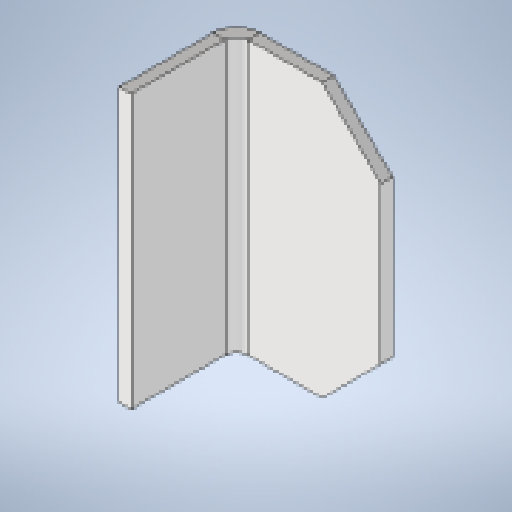
# Autodesk Inventor part: PNS-0812 floor ring  strengthen
Saved by Autodesk Inventor 2025.1 (Build 291241020, 241B)
## iProperties
Created: 2024-05-23
Part Number: PNS-0812 floor ring  strengthen
Material: Generic
Document SubType Name: Sheet Metal
Designer: user
Mass: 0.559799 g
Surface Area: 23.3947 cm^2
Volume: 0.559799 cm^3
Density: 1 g/cm^3
Flat Pattern Width: 12.9572 cm
Flat Pattern Length: 14 cm
Flat Pattern Area: 181.4 cm^2
Sheet Metal Rule: Default_mm
Sheet Metal Width: 129.572 mm
Sheet Metal Length: 140.000 mm
Sheet Metal Area: 18140.035 mm^2
Appearance: Default
Author: admin
Autodesk Inventor part; units mm, degrees
ref_plane "YZ Plane" through (0, 0, 0) normal (1, 0, 0) x (0, 1, 0)
ref_plane "XZ Plane" through (0, 0, 0) normal (0, 1, 0) x (-1, 0, 0)
ref_plane "XY Plane" through (0, 0, 0) normal (0, 0, 1) x (1, 0, 0)
sketch "Sketch1" plane through (0, 0, 0) normal (0, 0, 1) x (1, 0, 0)
  line L0 (0, 70) -> (80, 70)
  line L1 (80, 70) -> (80, -70)
  line L2 (80, -70) -> (0, -70)
  line L3 (0, -70) -> (0, 70)
  line L4 (40, 70) -> (40, -70) construction
  line L5 (50, 70) -> (80, 40)
  line L6 (80, -40) -> (50, -70)
  point P0 (0, 0)
  point P1 (0, 0)
  dimension "d1" = 140
  dimension "d15" = 30
  dimension "d27" = 80
  dimension "d28" = 45
  measures "d1" distance of L0.end L1.end
  measures "d15" distance of L0.end L5.start
  measures "d27" distance between parallel lines of L1 L3
  measures "d28" angle of L2 L6
extrude "Plate1" add sketch "Sketch1" along normal blind 6 contours L0 L5 L1 L6 L2 L3
sketch "Sketch3" plane through (6, -70, 0) normal (-1, 0, 0) x (0, -1, 0)
  line L0 (-140, 0) -> (0, 0)
  line L1 (0, 0) -> (0, 60)
  line L2 (0, 60) -> (-140, 60)
  line L3 (-140, 60) -> (-140, 0)
  constraints: 6 end point, 1 horizontal, 1 perpendicular, 1 vertical
edge flange "Flange1" height 60 angle 90 thickness 6 bend radius 6 thickness toward (-1, 0, 0) relief tear relief width 6 relief depth 3 edges at (0, 0, 6) wall of the first edge with corners at (6, 70, 0) (6, -70, 0) (6, -70, 60) (6, 70, 60)
bend "Bend1"
corner "Corner1"
equation "\"d2\" = Thickness"
equation "\"d17\" = BendReliefWidth"
equation "\"d18\" = BendReliefDepth"
equation "\"d19\" = MinimumRemnant"
equation "\"d20\" = TransitionRadius"
equation "\"d23\" = BendRadius"
equation "\"d24\" = CornerReliefSize"
equation "\"d25\" = GapSize"
equation "\"d26\" = JacobiRadiusSize"
equation "\"BendRadius\" = Thickness"
equation "\"BendReliefWidth\" = Thickness"
equation "\"BendReliefDepth\" = 0.5 * Thickness"
equation "\"CornerReliefSize\" = 4 * Thickness"
equation "\"MinimumRemnant\" = 2 * Thickness"
equation "\"TransitionRadius\" = BendRadius"
equation "\"JacobiRadiusSize\" = BendRadius"
equation "\"GapSize\" = Thickness"
equation "\"Thickness\" = 6"
body "Solid1"
